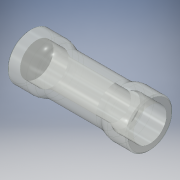
# Autodesk Inventor part: Axle-Connector
Saved by Autodesk Inventor 2016 (Build 200138000, 138)
## iProperties
Created: 2015-05-18
Part Number: Axle-Connector
Material: Generic
Document SubType Name: Modeling
Designer: jonathan
Density: 1 g/cm^3
Appearance: Clear
Mass: 0.647469 g
Surface Area: 10.5511 cm^2
Volume: 0.647469 cm^3
Author: jonathan
Autodesk Inventor part; units mm, degrees
ref_plane "XZ Plane" through (0, 0, 0) normal (0, 1, 0) x (-1, 0, 0)
ref_plane "Work Plane1" through (5.08, 0, 0) normal (1, 0, 0) x (0, 1, 0)
sketch "Sketch2" plane through (5.08, 0, 0) normal (1, 0, 0) x (0, 1, 0)
  circle A0 centre (0, 0) radius 3.81
  dimension "d2" = 7.62
  constraints: 1 centre point, 1 coincident
  measures "d2" diameter of A0
extrude "Extrusion1" add sketch "Sketch2" along normal blind 5.715
ref_plane "Work Plane2" through (3.81, 0, 0) normal (1, 0, 0) x (0, 1, 0)
sketch "Sketch3" plane through (3.81, 0, 0) normal (1, 0, 0) x (0, 1, 0)
  circle A0 centre (0, 0) radius 4.445
  dimension "d6" = 8.89
  constraints: 1 centre point, 1 coincident
  measures "d6" diameter of A0
loft "Loft1" add profiles "Sketch3" section 2 edges at (5.08, -3.81, 0)
extrude "Extrusion2" add sketch "Sketch3" against normal blind 4.445
mirror "Mirror1" about plane through (10.795, 0, 0) normal (1, 0, 0) of "Extrusion1", "Loft1", "Extrusion2"
shell "Shell1" thickness 1.27 removed faces 1 at (22.225, 1.6691, 0.6886)
fillet "Fillet1" radius 3.175 6 edges at (3.81, -4.445, 0) (5.08, -3.81, 0) (16.51, -3.81, 0) (17.78, -4.445, 0) (4.7802, -2.54, 0) (16.8098, -2.54, 0)
chamfer "Chamfer1" distance 0.254 angle 45 2 edges at (-0.635, -4.445, 0) (22.225, -4.445, 0)
body "Solid1"
